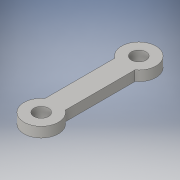
# Autodesk Inventor part: conneectors
Saved by Autodesk Inventor 2016 (Build 200138000, 138)
## iProperties
Created: 2016-05-25
Part Number: conneectors
Material: Generic
Document SubType Name: Modeling
Designer: jregalado
Density: 1 g/cm^3
Appearance: Default
Author: jregalado
Autodesk Inventor part; units mm, degrees
ref_plane "YZ Plane" through (0, 0, 0) normal (1, 0, 0) x (0, 1, 0)
ref_plane "XZ Plane" through (0, 0, 0) normal (0, 1, 0) x (-1, 0, 0)
ref_plane "XY Plane" through (0, 0, 0) normal (0, 0, 1) x (1, 0, 0)
sketch "Sketch1" plane through (0, 0, 0) normal (0, 1, 0) x (-1, 0, 0)
  line L0 (2.54, 10.414) -> (-2.54, 10.414)
  line L1 (-2.54, 10.414) -> (-2.54, -10.414)
  line L2 (-2.54, -10.414) -> (2.54, -10.414)
  line L3 (2.54, -10.414) -> (2.54, 10.414)
  circle A0 centre (0, 12.2555) radius 1.8415
  circle A1 centre (0, -12.2555) radius 1.8415
  circle A2 centre (0, -12.2555) radius 4.318
  circle A3 centre (0, 12.2555) radius 4.318
  point P0 (0, 0)
  point P1 (0, 10.414)
  point P2 (0, -10.414)
  dimension "d6" = 3.683
  dimension "d0" = 10.414
  dimension "d1" = 20.828
  dimension "d2" = 10.414
  dimension "d3" = 5.08
  dimension "d4" = 2.54
  dimension "d5" = 2.54
  dimension "d7" = 8.636
  constraints: 8 end point, 2 centre point, 2 coincident, 2 midpoint, 2 parallel, 2 vertical alignment, 1 equal radius, 1 horizontal, 1 perpendicular, 4 other
  measures "d0" distance from line of L2 point (0, 0)
  measures "d1" distance between parallel lines of L2 L0
  measures "d2" distance from line of L0 point (0, 0)
  measures "d3" distance between parallel lines of L3 L1
  measures "d4" distance from line of L3 point (0, 0)
  measures "d5" distance from line of L1 point (0, 0)
  measures "d7" diameter of A2
extrude "Extrusion1" add sketch "Sketch1" along normal blind 1.27 and the other way blind 1.27
equation "\"d0\" = d2"
equation "\"d4\" = d5"
body "Solid1"
